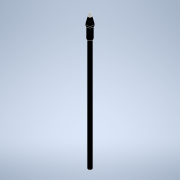
# Autodesk Inventor part: Ink Barrel + Tip
Saved by Autodesk Inventor 2021 (Build 250183000, 183)
## iProperties
Created: 2020-03-16
Part Number: Ink Barrel + Tip
Material: Generic
Document SubType Name: Modeling
Designer: Daniel
Density: 1 g/cm^3
Appearance: Black
Author: Daniel
Autodesk Inventor part; units mm, degrees
ref_plane "YZ Plane" through (0, 0, 0) normal (1, 0, 0) x (0, 1, 0)
ref_plane "XZ Plane" through (0, 0, 0) normal (0, 1, 0) x (-1, 0, 0)
ref_plane "XY Plane" through (0, 0, 0) normal (0, 0, 1) x (1, 0, 0)
sketch "Sketch1" plane through (0, 0, 0) normal (0, 0, 1) x (1, 0, 0)
  line L0 (0, 0.1624) -> (0, 12.1749)
  line L1 (0, 12.1749) -> (1.524, 12.1749)
  line L2 (1.524, 12.1749) -> (1.524, 101.0749)
  line L3 (1.524, 101.0749) -> (0, 101.0749)
  line L4 (0, 101.0749) -> (0, 12.1749)
  line L5 (0, 101.0749) -> (1.9875, 101.0749)
  line L6 (1.9875, 101.0749) -> (1.9875, 110.2189)
  line L7 (1.9875, 110.2189) -> (0, 110.2189)
  line L8 (0, 110.2189) -> (0, 101.0749)
  line L9 (0, 110.2189) -> (2.54, 110.2189)
  line L10 (2.54, 110.2189) -> (2.54, 111.4889)
  line L11 (2.54, 111.4889) -> (0, 111.4889)
  line L12 (0, 111.4889) -> (0, 110.2189)
  line L13 (2.54, 111.4889) -> (1.27, 116.5689)
  line L14 (0, 116.5689) -> (0, 111.4889)
  line L15 (0, 116.5689) -> (1.27, 116.5689)
  line L16 (1.143, 116.5689) -> (0.6099, 119.3321)
  line L17 (0, 119.7439) -> (0, 116.5689)
  line L18 (0, 119.7439) -> (0.1111, 119.7439)
  arc A0 (0.6099, 119.3321) -> (0.1111, 119.7439) centre (0.1111, 119.2359) ccw
  point P0 (0, 0)
  point P1 (0.5305, 119.7439)
  dimension "d0" = 1.524
  dimension "d1" = 88.9
  dimension "d2" = 1.9875
  dimension "d3" = 9.144
  dimension "d4" = 2.54
  dimension "d5" = 1.27
  dimension "d6" = 5.08
  dimension "d7" = 1.27
  dimension "d8" = 1.143
  dimension "d9" = 3.175
  dimension "d10" = 0.508
  constraints: 38 end point, 6 parallel, 4 horizontal, 4 perpendicular, 3 point on line, 3 vertical, 2 point on circle, 2 tangent, 1 centre point
  measures "d0" distance of L0.end L1.end
  measures "d1" distance of L1.end L2.end
  measures "d2" distance of L3.end L5.end
  measures "d3" distance of L5.end L6.end
  measures "d4" distance of L10.end L11.end
  measures "d5" distance of L9.end L10.end
  measures "d6" vertical distance of L10.end L13.end
  measures "d7" distance of L13.end L14.start
  measures "d8" distance of L16.start L14.start
  measures "d9" vertical distance of L16.start point (0.531, 119.744)
  measures "d10" radius of A0
revolve "Revolution1" add sketch "Sketch1" angle 360 about axis through (0, 119.7439, 0) along (0, -1, 0)
body "Solid1"
